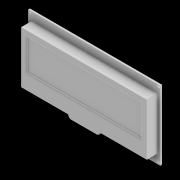
# Autodesk Inventor part: oscilloscope-screen
Saved by Autodesk Inventor 2020 (Build 240168000, 168)
## iProperties
Created: 2020-01-13
Part Number: oscilloscope-screen
Material: Generic
Document SubType Name: Modeling
Designer: valer
Density: 1 g/cm^3
Appearance: Default
Author: valer
Autodesk Inventor part; units mm, degrees
ref_plane "YZ Plane" through (0, 0, 0) normal (1, 0, 0) x (0, 1, 0)
ref_plane "XZ Plane" through (0, 0, 0) normal (0, 1, 0) x (-1, 0, 0)
ref_plane "XY Plane" through (0, 0, 0) normal (0, 0, 1) x (1, 0, 0)
sketch "TopProfile" plane through (0, 0, 0) normal (0, 0, 1) x (1, 0, 0)
  line L0 (0, 0) -> (66.675, 0)
  line L1 (66.675, 0) -> (66.675, 34.925)
  line L2 (66.675, 34.925) -> (0, 34.925)
  line L3 (0, 34.925) -> (0, 0)
  line L4 (1.5875, 30.5594) -> (65.0875, 30.5594)
  line L5 (65.0875, 30.5594) -> (65.0875, 4.3656)
  line L6 (65.0875, 4.3656) -> (1.5875, 4.3656)
  line L7 (1.5875, 4.3656) -> (1.5875, 30.5594)
  line L8 (25.4, 4.3656) -> (41.275, 4.3656)
  line L9 (41.275, 4.3656) -> (41.275, 2.7781)
  line L10 (41.275, 2.7781) -> (25.4, 2.7781)
  line L11 (25.4, 2.7781) -> (25.4, 4.3656)
  line L12 (4.3656, 27.7812) -> (62.3094, 27.7812)
  line L13 (62.3094, 27.7812) -> (62.3094, 11.9063)
  line L14 (62.3094, 11.9063) -> (4.3656, 11.9062)
  line L15 (4.3656, 11.9062) -> (4.3656, 27.7812)
  point P0 (33.3375, 4.3656)
  dimension "d0" = 66.675
  dimension "d1" = 34.925
  dimension "d2" = 26.1938
  dimension "d3" = 63.5
  dimension "d4" = 1.5875
  dimension "d5" = 1.6002
  dimension "d6" = 27.7812
  dimension "d7" = 15.875
  dimension "d8" = 4.3656
  dimension "d9" = 15.875
  dimension "d10" = 2.7781
  dimension "d11" = 2.7781
  dimension "d12" = 2.7781
  constraints: 32 end point, 8 parallel, 4 horizontal, 4 perpendicular, 2 midpoint, 1 point on line
  measures "d0" distance of L1.end L2.end
  measures "d1" distance of L2.end L0.start
  measures "d2" distance of L4.end L5.end
  measures "d3" distance of L4.start L4.end
  measures "d4" distance between parallel lines of L3 L7
  measures "d6" distance between parallel lines of L10 L4
  measures "d7" distance of L9.end L10.end
  measures "d8" distance between parallel lines of L2 L4
  measures "d9" distance of L12.end L13.end
  measures "d10" distance between parallel lines of L7 L15
  measures "d11" distance between parallel lines of L5 L13
  measures "d12" distance between parallel lines of L4 L12
extrude "BoardFeature" add sketch "TopProfile" against normal blind 0.7937 contours L3 L2 L1 L0 | L4 L5 L6 L7 | L6 L9 L10 L11 | L12 L13 L14 L15
extrude "ScreenFeature" add sketch "TopProfile" along normal blind 5.1594 contours L4 L5 L6 L7 | L6 L9 L10 L11
extrude "DisplayFeature" add sketch "TopProfile" along normal blind 4.572 contours L12 L13 L14 L15
fillet "BezelFilletsFeature" radius 0.254 4 edges at (4.3656, 27.7812, 4.8657) (62.3094, 27.7812, 4.8657) (62.3094, 11.9063, 4.8657) (4.3656, 11.9062, 4.8657)
fillet "BottomFilletsFeature" radius 1.524 2 edges at (25.4, 2.7781, 2.5797) (41.275, 2.7781, 2.5797)
sketch "MountHoles" plane through (0, 0, 0) normal (0, 0, 1) x (1, 0, 0)
  circle A0 centre (0.7937, 0.7937) radius 0.7937
  circle A1 centre (65.8813, 0.7937) radius 0.7937
  line L0 (0, 0) -> (66.675, 0) construction
  line L1 (0, 34.925) -> (0, 0) construction
  line L2 (66.675, 0) -> (66.675, 34.925) construction
  circle A2 centre (0.7937, 34.1313) radius 0.7937
  circle A3 centre (65.8812, 34.1313) radius 0.7937
  line L3 (66.675, 34.925) -> (0, 34.925) construction
  dimension "d21" = 1.5875
  dimension "d32" = 65.0875
  constraints: 8 tangent, 4 centre point, 3 equal radius
  measures "d21" diameter of A0
  measures "d32" distance of A1.centre A0.centre
hole "MountHolesFeature" at (0.7937, 0.7937, 0) at (0.7937, 34.1313, 0) at (65.8812, 34.1313, 0) at (65.8813, 0.7937, 0) direction (0, 0, -1) diameter 1.27 end through all
equation "\"d11\" = d10"
equation "\"d12\" = d10"
body "Solid1"
